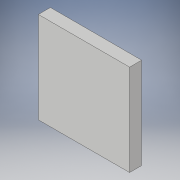
# Autodesk Inventor part: Convex Organ Bank Brain Slot
Saved by Autodesk Inventor 2019 (Build 230136000, 136)
## iProperties
Created: 2021-02-18
Part Number: Convex Organ Bank Brain Slot
Material: Generic
Document SubType Name: Modeling
Designer: Eric
Density: 1 g/cm^3
Appearance: Default
Author: Eric
Autodesk Inventor part; units mm, degrees
ref_plane "YZ Plane" through (0, 0, 0) normal (1, 0, 0) x (0, 1, 0)
ref_plane "XZ Plane" through (0, 0, 0) normal (0, 1, 0) x (-1, 0, 0)
ref_plane "XY Plane" through (0, 0, 0) normal (0, 0, 1) x (1, 0, 0)
sketch "Sketch1" plane through (0, 0, 0) normal (0, 0, 1) x (1, 0, 0)
  line L0 (7.5, -7.5) -> (98.5, -7.5) construction
  line L1 (98.5, -7.5) -> (98.5, -98.5) construction
  line L2 (98.5, -98.5) -> (7.5, -98.5) construction
  line L3 (7.5, -98.5) -> (7.5, -7.5) construction
  line L4 (0, 0) -> (106, 0)
  line L5 (106, 0) -> (106, -106)
  line L6 (106, -106) -> (0, -106)
  line L7 (0, -106) -> (0, 0)
  dimension "d0" = 91
  dimension "d1" = 91
  dimension "d2" = 7.5
  dimension "d3" = 7.5
  dimension "d5" = 7.5
  dimension "d6" = 7.5
  constraints: 16 end point, 3 horizontal, 3 vertical
  measures "d0" distance of L1.end L2.end
  measures "d1" distance of L0.end L1.end
  measures "d2" distance between parallel lines of L7 L3
  measures "d3" distance between parallel lines of L4 L0
  measures "d5" distance between parallel lines of L5 L1
  measures "d6" distance between parallel lines of L2 L6
extrude "Extrusion1" add sketch "Sketch1" along normal blind 14
equation "\"d3\" = d2"
equation "\"d5\" = d3"
equation "\"d6\" = d3"
body "Solid1"
